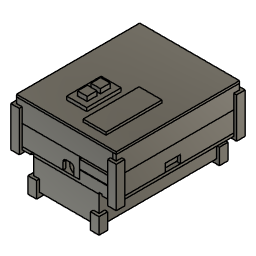
Thermocycler_build v6 (Autodesk Fusion 360 design; units mm, degrees)
Autodesk Fusion 360 part; units mm, degrees
(part 1 of 2)
sketch "Sketch1" plane through (0, 0, 0) normal (0, 0, 1) x (1, 0, 0)
  line L0 (0, 0) -> (114, 0)
  line L1 (114, 0) -> (114, 215)
  line L2 (114, 215) -> (0, 215)
  line L3 (0, 215) -> (0, 0)
  dimension "d1" = 114
  dimension "d2" = 215
  constraint horizontal L0
  constraint vertical L1
  constraint horizontal L2
  constraint vertical L3
  constraint coincident L0.start L3.end
  measures "d1" distance of L0.start L0.end
  measures "d2" distance of L0.start L2.end
extrude "Extrude1" add sketch "Sketch1" along normal blind 49 makes body 1
sketch "Sketch2" plane through (0, 0, 0) normal (0, 0, 1) x (1, 0, 0)
  line L0 (0, 0) -> (50, 0)
  line L1 (50, 0) -> (50, 138)
  line L2 (50, 138) -> (0, 138)
  line L3 (0, 138) -> (0, 0)
  dimension "d5" = 50
  dimension "d6" = 138
  constraint horizontal L0
  constraint vertical L1
  constraint horizontal L2
  constraint vertical L3
  constraint coincident L0.start L3.end
  measures "d5" distance of L0.start L0.end
  measures "d6" distance of L0.start L2.end
extrude "Extrude2" add sketch "Sketch2" along normal blind 21 separate body makes body 2
copy_body "Body->Comp1" bodies 1 removing the originals makes body 3 in component "Alimentatore"
copy_body "Body->Comp2" bodies 2 removing the originals makes body 4 in component "Relays"
sketch "Sketch3" plane through (0, 0, 0) normal (0, 0, 1) x (1, 0, 0)
  line L0 (0, 0) -> (26, 0)
  line L1 (26, 0) -> (26, 50)
  line L2 (26, 50) -> (0, 50)
  line L3 (0, 50) -> (0, 0)
  dimension "d9" = 26
  dimension "d10" = 50
  constraint horizontal L0
  constraint vertical L1
  constraint horizontal L2
  constraint vertical L3
  constraint coincident L0.start L3.end
  measures "d9" distance of L0.start L0.end
  measures "d10" distance of L0.start L2.end
extrude "Extrude3" add sketch "Sketch3" along normal blind 15 separate body makes body 5
copy_body "Body->Comp3" bodies 5 removing the originals makes body 6 in component "Buck_conv"
sketch "Sketch4" plane through (0, 0, 0) normal (0, 0, 1) x (1, 0, 0)
  line L0 (0, 0) -> (82, 0)
  line L1 (82, 0) -> (82, 54)
  line L2 (82, 54) -> (0, 54)
  line L3 (0, 54) -> (0, 0)
  dimension "d13" = 82
  dimension "d14" = 54
  constraint horizontal L0
  constraint vertical L1
  constraint horizontal L2
  constraint vertical L3
  constraint coincident L0.start L3.end
  measures "d13" distance of L0.start L0.end
  measures "d14" distance of L0.start L2.end
extrude "Extrude4" add sketch "Sketch4" along normal blind 10 separate body makes body 7
copy_body "Body->Comp4" bodies 7 removing the originals makes body 8 in component "Breadbord"
sketch "Sketch5" plane through (0, 0, 0) normal (0, 0, 1) x (1, 0, 0)
  line L0 (0, 0) -> (58, 0)
  line L1 (58, 0) -> (58, 82)
  line L2 (58, 82) -> (0, 82)
  line L3 (0, 82) -> (0, 0)
  dimension "d17" = 58
  dimension "d18" = 82
  constraint horizontal L0
  constraint vertical L1
  constraint horizontal L2
  constraint vertical L3
  constraint coincident L0.start L3.end
  measures "d17" distance of L0.start L0.end
  measures "d18" distance of L0.start L2.end
extrude "Extrude5" add sketch "Sketch5" along normal blind 15 separate body makes body 9
copy_body "Body->Comp5" bodies 9 removing the originals makes body 10 in component "Arduino"
sketch "Sketch6" plane through (0, 0, 0) normal (0, 0, 1) x (1, 0, 0)
  line L0 (0, 0) -> (18, 0)
  line L1 (18, 0) -> (18, 35)
  line L2 (18, 35) -> (0, 35)
  line L3 (0, 35) -> (0, 0)
  dimension "d21" = 18
  dimension "d22" = 35
  constraint horizontal L0
  constraint vertical L1
  constraint horizontal L2
  constraint vertical L3
  constraint coincident L0.start L3.end
  measures "d21" distance of L0.start L0.end
  measures "d22" distance of L0.start L2.end
extrude "Extrude6" add sketch "Sketch6" along normal blind 15 separate body makes body 11
copy_body "Body->Comp6" bodies 11 removing the originals makes body 12 in component "Mosfet"
sketch "Sketch7" plane through (0, 0, 0) normal (0, 0, 1) x (1, 0, 0)
  line L0 (0, 0) -> (40, 0)
  line L1 (40, 0) -> (40, 73)
  line L2 (40, 73) -> (0, 73)
  line L3 (0, 73) -> (0, 0)
  dimension "d25" = 40
  dimension "d26" = 73
  constraint horizontal L0
  constraint vertical L1
  constraint horizontal L2
  constraint vertical L3
  constraint coincident L0.start L3.end
  measures "d25" distance of L0.start L0.end
  measures "d26" distance of L0.start L2.end
extrude "Extrude7" add sketch "Sketch7" along normal blind 24 separate body makes body 13
copy_body "Body->Comp7" bodies 13 removing the originals makes body 14 in component "Big_relay"
copy_body "CopyPasteBodies1" bodies 12 makes body 15 in component "Mosfet"
move_body "Move1" bodies 15 to x (1, 0, 0) y (0, 1, 0) z (0, 0, 1) at (-20, 20, 0) in component "Mosfet"
move_body "Move2" bodies 12 to x (1, 0, 0) y (0, 1, 0) z (0, 0, 1) at (4, 0, 0) in component "Mosfet"
copy_body "CopyPasteBodies2" bodies 12 makes body 16 in component "Mosfet"
move_body "Move3" bodies 16 to x (1, 0, 0) y (0, 1, 0) z (0, 0, 1) at (0, 60, 0) in component "Mosfet"
sketch "Sketch8" plane through (0, 0, 49) normal (0, 0, 1) x (-1, 0, 0)
  line L0 (0, -215) -> (0, 0)
  line L1 (0, 0) -> (-114, 0)
  line L2 (-114, 0) -> (-114, -215)
  line L3 (-114, -215) -> (0, -215)
  line L4 (-144, 30) -> (-144, -245)
  line L5 (-144, -245) -> (30, -245)
  line L6 (30, -245) -> (30, 30)
  line L7 (30, 30) -> (-144, 30)
  line L8 (0, -215) -> (30, -215)
  line L9 (-114, -215) -> (-144, -215)
  line L10 (-114, 0) -> (-144, 0)
  line L11 (0, 0) -> (30, 0)
  line L12 (20, -203) -> (-30, -203)
  line L13 (-30, -203) -> (-30, -65)
  line L14 (-30, -65) -> (20, -65)
  line L15 (20, -65) -> (20, -203)
  line L16 (21.5, -51.5) -> (-51.5, -51.5)
  line L17 (-51.5, -51.5) -> (-51.5, -11.5)
  line L18 (-51.5, -11.5) -> (21.5, -11.5)
  line L19 (21.5, -11.5) -> (21.5, -51.5)
  line L20 (-36, -150) -> (-54, -150)
  line L21 (-54, -150) -> (-54, -115)
  line L22 (-54, -115) -> (-36, -115)
  line L23 (-36, -115) -> (-36, -150)
  line L24 (-60, -190) -> (-78, -190)
  line L25 (-78, -190) -> (-78, -155)
  line L26 (-78, -155) -> (-60, -155)
  line L27 (-60, -155) -> (-60, -190)
  line L28 (-36, -210) -> (-54, -210)
  line L29 (-54, -210) -> (-54, -175)
  line L30 (-54, -175) -> (-36, -175)
  line L31 (-36, -175) -> (-36, -210)
  line L32 (-88, -203) -> (-138, -203)
  line L33 (-138, -203) -> (-138, -177)
  line L34 (-138, -177) -> (-88, -177)
  line L35 (-88, -177) -> (-88, -203)
  line L36 (-84, -173) -> (-138, -173)
  line L37 (-138, -173) -> (-138, -91)
  line L38 (-138, -91) -> (-84, -91)
  line L39 (-84, -91) -> (-84, -173)
  line L40 (-80, -82) -> (-138, -82)
  line L41 (-138, -82) -> (-138, 0)
  line L42 (-138, 0) -> (-80, 0)
  line L43 (-80, 0) -> (-80, -82)
  line L44 (0, -215) -> (-114, -215)
  line L45 (-114, -215) -> (-114, 0)
  line L46 (-114, 0) -> (0, 0)
  line L47 (0, 0) -> (0, -215)
  line L48 (-114, 0) -> (-77, 0) construction
  line L49 (-77, 0) -> (-77, -44) construction
  line L50 (-77, -44) -> (-114, -44) construction
  line L51 (-114, -44) -> (-114, 0) construction
  circle A0 centre (-77, -44) radius 32.5
  line L52 (-80, 0) -> (-138, 0)
  line L53 (-138, 0) -> (-138, -9)
  line L54 (-138, -9) -> (-80, -9)
  line L55 (-80, -9) -> (-80, 0)
  line L56 (-138, -82) -> (-118, -82)
  line L57 (-118, -82) -> (-118, -72)
  line L58 (-118, -72) -> (-138, -72)
  line L59 (-138, -72) -> (-138, -82)
  dimension "d29" = 30
  dimension "d30" = 37
  dimension "d31" = 44
  dimension "d32" = 65
  dimension "d33" = 58
  dimension "d34" = 9
  dimension "d35" = 20
  dimension "d36" = 10
  constraint coincident L0.start L3.end
  constraint coincident L6 L8.end
  constraint perpendicular L6 L8
  constraint coincident L2.end L3.start
  constraint coincident L4 L9.end
  constraint perpendicular L4 L9
  constraint coincident L1.end L2.start
  constraint coincident L4 L10.end
  constraint perpendicular L4 L10
  constraint coincident L0.end L1.start
  constraint coincident L6 L11.end
  constraint perpendicular L6 L11
  constraint horizontal L12
  constraint vertical L13
  constraint horizontal L14
  constraint vertical L15
  constraint horizontal L16
  constraint vertical L17
  constraint horizontal L18
  constraint vertical L19
  constraint horizontal L20
  constraint vertical L21
  constraint horizontal L22
  constraint vertical L23
  constraint horizontal L24
  constraint vertical L25
  constraint horizontal L26
  constraint vertical L27
  constraint horizontal L28
  constraint vertical L29
  constraint horizontal L30
  constraint vertical L31
  constraint horizontal L32
  constraint vertical L33
  constraint horizontal L34
  constraint vertical L35
  constraint horizontal L36
  constraint vertical L37
  constraint horizontal L38
  constraint vertical L39
  constraint horizontal L40
  constraint vertical L41
  constraint horizontal L42
  constraint vertical L43
  constraint horizontal L44
  constraint vertical L45
  constraint horizontal L46
  constraint vertical L47
  constraint horizontal L48
  constraint vertical L49
  constraint horizontal L50
  constraint vertical L51
  constraint coincident L49.end L50.start
  constraint horizontal L52
  constraint vertical L53
  constraint horizontal L54
  constraint vertical L55
  constraint horizontal L56
  constraint vertical L57
  constraint horizontal L58
  constraint vertical L59
  measures "d30" distance of L1.end L48.end
  measures "d31" distance of L1.end L50.end
  measures "d32" diameter of A0
  measures "d33" distance of L42.end L41.end
  measures "d34" distance of L42.end L54.end
  measures "d35" distance of L40.end L56.end
  measures "d36" distance of L40.end L58.end
extrude "Extrude1'" add sketch "Sketch8" along normal blind 5 separate body contours L0 L2 L3 L12 L13 L14 L16 L32 L34 L35 L36 L38 L39 L40 L43 L44 L45 L47 A0 | L0 L6 L8 L11 L12 L14 L15 L16 L18 L19 L47 | L0 L12 L13 L14 L47 | L0 L12 L14 L15 L47 | L2 L4 L9 L10 L32 L33 L34 L36 L37 L38 L40 L41 L45 L53 L56 L59 | L2 L32 L33 L34 L45 | L2 L32 L34 L35 L45 | L0 L16 L17 L18 L47 A0 | L0 L16 L18 L19 L47 | L0 L1 L17 L18 L43 L46 L47 A0 L55 | L2 L36 L37 L38 L45 | L2 L36 L38 L39 L45 | L2 L10 L41 L42 L45 L52 L53 L54 | L1 L2 L42 L43 L45 L46 L52 L54 L55 | L2 L40 L43 L45 A0 L54 | L2 L40 L41 L45 L54 L57 L58 | L40 L41 L56 L57 L58 L59 | L20 L21 L22 L23 | L24 L25 L26 L27 | L28 L29 L30 L31 makes body 17 in component "Alimentatore"
copy_body "CutPasteBodies1" bodies 17 removing the originals makes body 18
extrude "Extrude8" add sketch "Sketch8" along normal blind 20 contours L2 L10 L41 L42 L45 L52 L53 L54 | L1 L2 L42 L43 L45 L46 L52 L54 L55 | L40 L41 L56 L57 L58 L59 bodies 18
fillet "Fillet1" radius 10 1 edges at (107.3006, 32.2475, 54) on bodies 18
sketch "Sketch9" plane through (0, 0, 54) normal (0, 0, 1) x (-1, 0, 0)
  arc A0 (-98.6603, -9) -> (-80, -2.9492) centre (-77, -44) ccw
  line L0 (-98.6603, -9) -> (-138, -9)
  line L1 (-138, -9) -> (-138, 0)
  line L2 (-138, 0) -> (-144, 0)
  line L3 (-144, 0) -> (-144, -215)
  line L4 (-144, -215) -> (30, -215)
  line L5 (30, -215) -> (30, 0)
  line L6 (30, 0) -> (-80, 0)
  line L7 (-80, 0) -> (-80, -2.9492)
  line L8 (-138, -72) -> (-118, -72)
  line L9 (-118, -72) -> (-118, -82)
  line L10 (-118, -82) -> (-138, -82)
  line L11 (-138, -82) -> (-138, -72)
  line L12 (-144, -215) -> (-114, -215) construction
  line L13 (30, -215) -> (0, -215) construction
  line L14 (-114, -215) -> (0, -215) construction
  line L15 (0, -215) -> (0, -195)
  line L16 (0, -195) -> (-114, -195)
  line L17 (-114, -195) -> (-114, -215)
  line L18 (-57, -195) -> (-57, -185) construction
  line L19 (-57, -185) -> (-47, -185) construction
  line L20 (-47, -185) -> (-22, -185) construction
  line L21 (-22, -185) -> (-47, -185)
  line L22 (-47, -185) -> (-47, -153)
  line L23 (-47, -153) -> (-22, -153)
  line L24 (-22, -153) -> (-22, -185)
  line L25 (-57, -185) -> (-82, -185)
  line L26 (-82, -185) -> (-82, -153)
  line L27 (-82, -153) -> (-57, -153)
  line L28 (-57, -153) -> (-57, -185)
  dimension "d43" = 30
  dimension "d44" = 30
  dimension "d45" = 20
  dimension "d46" = 10
  dimension "d47" = 10
  dimension "d48" = 25
  dimension "d49" = 25
  dimension "d50" = 32
  dimension "d51" = 25
  dimension "d52" = 32
  constraint coincident L3.end L4.start
  constraint perpendicular L3 L12
  constraint coincident L4.end L5.start
  constraint perpendicular L5 L13
  constraint horizontal L14
  constraint vertical L15
  constraint horizontal L16
  constraint vertical L17
  constraint midpoint L16 L18.start
  constraint perpendicular L16 L18
  constraint perpendicular L18 L19
  constraint parallel L19 L20
  constraint horizontal L21
  constraint vertical L22
  constraint horizontal L23
  constraint vertical L24
  constraint coincident L13.end L15
  constraint horizontal L25
  constraint vertical L26
  constraint horizontal L27
  constraint vertical L28
  measures "d43" distance of L3.end L12.end
  measures "d44" distance of L4.end L13.end
  measures "d45" distance of L12.end L16.end
  measures "d46" distance of L18.start L18.end
  measures "d47" distance of L18.end L19.end
  measures "d48" distance of L19.end L20.end
  measures "d49" distance of L20.end L19.end
  measures "d50" distance of L20.end L23.end
  measures "d51" distance of L18.end L25.end
  measures "d52" distance of L18.end L27.end
extrude "Extrude9" cut sketch "Sketch9" against normal blind 30 contours L4 L15 L16 L17 | L21 L22 L23 L24 | L25 L26 L27 L28 bodies 18
move_body "Move4" bodies 15 to x (1, 0, 0) y (0, 1, 0) z (0, 0, 1) at (0, 20, 0) in component "Mosfet"
move_body "Move5" bodies 12 to x (1, 0, 0) y (0, 1, 0) z (0, 0, 1) at (0, 35, 0) in component "Mosfet"
move_body "Move6" bodies 16 to x (1, 0, 0) y (0, 1, 0) z (0, 0, 1) at (0, 15, 0) in component "Mosfet"
move_body "Move7" bodies 15 to x (1, 0, 0) y (0, 1, 0) z (0, 0, 1) at (0, -10, 0) in component "Mosfet"
sketch "Sketch10" plane through (0, 0, 54) normal (0, 0, 1) x (-1, 0, 0)
  line L0 (0, -195) -> (0, -215)
  line L1 (0, -215) -> (30, -215)
  line L2 (30, -215) -> (30, 0)
  line L3 (30, 0) -> (-80, 0)
  line L4 (-80, 0) -> (-80, -2.9492)
  arc A0 (-98.6603, -9) -> (-80, -2.9492) centre (-77, -44) ccw
  line L5 (-98.6603, -9) -> (-138, -9)
  line L6 (-138, -9) -> (-138, 0)
  line L7 (-138, 0) -> (-144, 0)
  line L8 (-144, 0) -> (-144, -215)
  line L9 (-144, -215) -> (-114, -215)
  line L10 (-114, -215) -> (-114, -195)
  line L11 (-114, -195) -> (0, -195)
  line L12 (-82, -185) -> (-82, -153)
  line L13 (-82, -153) -> (-57, -153)
  line L14 (-57, -153) -> (-57, -185)
  line L15 (-57, -185) -> (-82, -185)
  line L16 (-47, -185) -> (-47, -153)
  line L17 (-47, -153) -> (-22, -153)
  line L18 (-22, -153) -> (-22, -185)
  line L19 (-22, -185) -> (-47, -185)
  line L20 (-138, -72) -> (-118, -72)
  line L21 (-118, -72) -> (-118, -82)
  line L22 (-118, -82) -> (-138, -82)
  line L23 (-138, -82) -> (-138, -72)
  line L24 (0, -210) -> (25, -210)
  line L25 (25, -210) -> (25, -5)
  line L26 (25, -5) -> (-80, -5)
  line L27 (-138, -5) -> (-139, -5)
  line L28 (-139, -5) -> (-139, -210)
  line L29 (-139, -210) -> (-114, -210)
  line L30 (-138, -5) -> (-138, 0)
  line L31 (-114, -210) -> (-114, -215)
  line L32 (-114, -210) -> (0, -210)
  line L33 (-114, -215) -> (0, -215)
  line L34 (-80, -5) -> (-80, 0)
  dimension "d55" = -5
  dimension "d56" = -5
  constraint coincident L6.end L7.start
  constraint perpendicular L7 L30
  constraint coincident L9.end L10.start
  constraint perpendicular L9 L31
  constraint perpendicular L0 L32
  constraint coincident L0.end L1.start
  constraint coincident L3.end L4.start
  constraint perpendicular L3 L34
extrude "Extrude10" add sketch "Sketch10" along normal blind 35 separate body contours L0 L1 L2 L3 L4 A0 L24 L25 L26 L34 | L0 L10 L31 L32 L33 | L6 L7 L8 L9 L10 L27 L28 L29 L30 L31 | A0 L26 L34 makes body 19
extrude "Extrude11" add 1 faces at (37.9469, 1.6667, 89) along direction (0, 0, 1) blind 40 separate body on bodies 19 makes body 20
extrude "Extrude12" add 2 faces at (80, 0.9831, 102.3333) (80, 4.3164, 102.3333) along direction (1, 0, 0) blind 60 on bodies 20 bodies 20
sketch "Sketch11" plane through (0, 0, 0) normal (0, 0, 1) x (1, 0, 0)
  line L0 (0, 0) -> (100, 0)
  line L1 (100, 0) -> (100, 60)
  line L2 (100, 60) -> (0, 60)
  line L3 (0, 60) -> (0, 0)
  line L4 (98.75, 10.1) -> (1.25, 10.1)
  line L5 (1.25, 10.1) -> (1.25, 49.9)
  line L6 (1.25, 49.9) -> (98.75, 49.9)
  line L7 (98.75, 49.9) -> (98.75, 10.1)
  line L8 (98.75, 10.1) -> (1.25, 49.9) construction
  line L9 (1.25, 10.1) -> (98.75, 49.9) construction
  point P0 (50, 30)
  dimension "d63" = 100
  dimension "d64" = 60
  dimension "d65" = 39.8
  dimension "d66" = 97.5
  dimension "d67" = 50
  dimension "d68" = 30
  constraint horizontal L0
  constraint vertical L1
  constraint horizontal L2
  constraint vertical L3
  constraint coincident L0.start L3.end
  constraint horizontal L4
  constraint perpendicular L4 L5
  constraint parallel L4 L6
  constraint parallel L5 L7
  constraint coincident L8 P0
  constraint coincident L9 P0
  measures "d63" distance of L0.start L0.end
  measures "d64" distance of L0.start L2.end
  measures "d65" distance of L4.end L5.end
  measures "d66" distance of L5.end L6.end
  measures "d67" distance of L1 P0
  measures "d68" distance of L2 P0
extrude "Extrude13" add sketch "Sketch11" along normal blind 2 separate body makes body 21
extrude "Extrude14" add sketch "Sketch11" along normal blind 10.5 contours L4 L5 L6 L7 bodies 21
move_body "Move1'" bodies 21 to x (0, -1, 0) y (1, 0, 0) z (0, 0, 1) at (-20, 110, 127)
sketch "Sketch12" plane through (0, 0, 129) normal (0, 0, 1) x (-1, 0, 0)
  line L0 (-138, -5) -> (25, -5)
  line L1 (25, -5) -> (25, -210)
  line L2 (25, -210) -> (-139, -210)
  line L3 (-139, -210) -> (-139, -5)
  line L4 (-139, -5) -> (-138, -5)
  line L5 (30, 0) -> (-138, 0)
  line L6 (-138, 0) -> (-144, 0)
  line L7 (-144, 0) -> (-144, -215)
  line L8 (-144, -215) -> (30, -215)
  line L9 (30, -215) -> (30, 0)
  line L10 (-144, 0) -> (30, 0)
  line L11 (30, 0) -> (30, -215)
  line L12 (30, -215) -> (-144, -215)
  line L13 (-144, -215) -> (-144, 0)
  line L14 (-119.9, -15) -> (-59.9, -15) construction
  line L15 (-59.9, -15) -> (-59.9, -115) construction
  line L16 (-59.9, -115) -> (-119.9, -115) construction
  line L17 (-119.9, -115) -> (-119.9, -15) construction
  line L18 (-119.9, -65) -> (-59.9, -65) construction
  line L19 (-89.9, -15) -> (-89.9, -115) construction
  line L20 (-69.9, -113.75) -> (-109.9, -113.75)
  line L21 (-109.9, -113.75) -> (-109.9, -16.25)
  line L22 (-109.9, -16.25) -> (-69.9, -16.25)
  line L23 (-69.9, -16.25) -> (-69.9, -113.75)
  line L24 (-69.9, -113.75) -> (-109.9, -16.25) construction
  line L25 (-109.9, -113.75) -> (-69.9, -16.25) construction
  point P0 (-89.9, -65)
  dimension "d73" = 40
  dimension "d74" = 97.5
  constraint horizontal L10
  constraint vertical L11
  constraint horizontal L12
  constraint vertical L13
  constraint coincident L8.end L9.start
  constraint coincident L6.end L7.start
  constraint horizontal L14
  constraint vertical L15
  constraint horizontal L16
  constraint vertical L17
  constraint midpoint L17 L18.start
  constraint midpoint L15 L18.end
  constraint midpoint L14 L19.start
  constraint midpoint L16 L19.end
  constraint horizontal L20
  constraint perpendicular L20 L21
  constraint parallel L20 L22
  constraint parallel L21 L23
  constraint coincident L24 P0
  constraint coincident L25 P0
  constraint midpoint L18 P0
  measures "d73" distance of L21.end L22.end
  measures "d74" distance of L20.end L21.end
extrude "Extrude15" add sketch "Sketch12" along normal blind 5 separate body contours L0 L1 L2 L3 L4 | L5 L6 L7 L8 L9 L10 L11 L12 L13 makes body 22
sketch "Sketch13" plane through (0, 0, 49) normal (0, 0, -1) x (1, 0, 0)
  circle A0 centre (77, -44) radius 32.5
  line L0 (0, -215) -> (0, -195)
  line L1 (0, -195) -> (114, -195)
  line L2 (114, -195) -> (114, -215)
  line L3 (114, -215) -> (144, -215)
  line L4 (144, -215) -> (144, 0)
  line L5 (144, 0) -> (-30, 0)
  line L6 (-30, 0) -> (-30, -215)
  line L7 (-30, -215) -> (0, -215)
  line L8 (47, -153) -> (47, -185)
  line L9 (47, -185) -> (22, -185)
  line L10 (22, -185) -> (22, -153)
  line L11 (22, -153) -> (47, -153)
  line L12 (82, -153) -> (82, -185)
  line L13 (82, -185) -> (57, -185)
  line L14 (57, -185) -> (57, -153)
  line L15 (57, -153) -> (82, -153)
  line L16 (0, 0) -> (-5, 0)
  line L17 (-5, 0) -> (-5, -215)
  line L18 (-5, -215) -> (0, -215)
  line L19 (0, -215) -> (0, 0)
  line L20 (114, 0) -> (119, 0)
  line L21 (119, 0) -> (119, -215)
  line L22 (119, -215) -> (114, -215)
  line L23 (114, -215) -> (114, 0)
  dimension "d77" = 5
  constraint horizontal L16
  constraint vertical L17
  constraint horizontal L18
  constraint vertical L19
  constraint coincident L7 L17.end
  constraint coincident L16.start L19.end
  constraint horizontal L20
  constraint vertical L21
  constraint horizontal L22
  constraint vertical L23
  constraint coincident L3 L21.end
  constraint coincident L5 L20.start
  measures "d77" distance of L20.start L20.end
extrude "Extrude16" cut sketch "Sketch13" against normal blind 2.5 contours L0 L5 L7 L16 L17 L18 L19 | L2 L3 L5 L20 L21 L22 L23 bodies 18
sketch "Sketch14" plane through (0, 0, 0) normal (0, -1, 0) x (1, 0, 0)
  line L0 (-30, 54) -> (80, 54)
  line L1 (80, 54) -> (80, 89)
  line L2 (80, 89) -> (-30, 89)
  line L3 (-30, 89) -> (-30, 54)
  line L4 (70, 54) -> (51, 54)
  line L5 (51, 54) -> (51, 66.5)
  line L6 (56.5, 72) -> (64.5, 72)
  line L7 (70, 66.5) -> (70, 54)
  arc A0 (56.5, 72) -> (51, 66.5) centre (56.5, 66.5) ccw
  arc A1 (70, 66.5) -> (64.5, 72) centre (64.5, 66.5) ccw
  point P0 (70, 72)
  dimension "d80" = 19
  dimension "d81" = 18
  dimension "d82" = 5.5
  constraint horizontal L4
  constraint vertical L5
  constraint horizontal L6
  constraint vertical L7
  constraint coincident L0 L4.start
  constraint tangent L5 A0
  constraint tangent L6 A0
  constraint coincident P0 L6
  constraint coincident P0 L7
  constraint tangent L6 A1
  constraint tangent L7 A1
  constraint equal A0 A1
  measures "d80" distance of L4.start L4.end
  measures "d81" distance of L4.start P0
  measures "d82" radius of A0
extrude "Extrude17" cut sketch "Sketch14" against normal blind 10 contours L0 L4 L5 L6 L7 A0 A1 bodies 19
sketch "Sketch15" plane through (144, 0, 0) normal (1, 0, 0) x (0, 1, 0)
  line L0 (0, 54) -> (215, 54)
  line L1 (215, 54) -> (215, 89)
  line L2 (215, 89) -> (0, 89)
  line L3 (0, 89) -> (0, 54)
  line L4 (0, 89) -> (82, 89)
  line L5 (82, 89) -> (82, 89)
  line L6 (82, 89) -> (0, 89)
  line L7 (0, 89) -> (0, 89)
  line L8 (82, 89) -> (85.5, 89) construction
  line L9 (85.5, 89) -> (85.5, 54) construction
  line L10 (85.5, 54) -> (112, 54)
  line L11 (112, 54) -> (112, 68)
  line L12 (112, 68) -> (85.5, 68)
  line L13 (85.5, 68) -> (85.5, 54)
  dimension "d85" = 3.5
  dimension "d86" = 26.5
  dimension "d87" = 14
  constraint horizontal L4
  constraint horizontal L6
  constraint coincident L2 L4.end
  constraint coincident L2.end L3.start
  constraint parallel L2 L8
  constraint coincident L0 L9.end
  constraint perpendicular L0 L9
  constraint horizontal L10
  constraint vertical L11
  constraint horizontal L12
  constraint vertical L13
  measures "d85" distance of L4.end L8.end
  measures "d86" distance of L9.end L10.end
  measures "d87" distance of L9.end L12.end
extrude "Extrude18" cut sketch "Sketch15" against normal blind 5 contours L0 L10 L11 L12 L13 bodies 19
sketch "Sketch16" plane through (0, 215, 0) normal (0, 1, 0) x (-1, 0, 0)
  line L0 (-144, 54) -> (30, 54)
  line L1 (30, 54) -> (30, 89)
  line L2 (30, 89) -> (-144, 89)
  line L3 (-144, 89) -> (-144, 54)
  circle A0 centre (-119.9965, 81.996) radius 2.5
  circle A1 centre (-105, 65) radius 2.5
  line L4 (-103.1254, 66.6541) -> (-118.1219, 83.6501)
  line L5 (-121.8711, 80.342) -> (-106.8746, 63.3459)
  circle A2 centre (-104.2822, 81.996) radius 2.5
  circle A3 centre (-89.2857, 65) radius 2.5
  line L6 (-106.1568, 80.342) -> (-91.1603, 63.3459)
  line L7 (-87.4111, 66.6541) -> (-102.4076, 83.6501)
  circle A4 centre (-88.5679, 81.996) radius 2.5
  circle A5 centre (-73.5714, 65) radius 2.5
  line L8 (-90.4425, 80.342) -> (-75.446, 63.3459)
  line L9 (-71.6968, 66.6541) -> (-86.6933, 83.6501)
  circle A6 centre (-72.8536, 81.996) radius 2.5
  circle A7 centre (-57.8571, 65) radius 2.5
  line L10 (-74.7282, 80.342) -> (-59.7317, 63.3459)
  line L11 (-55.9825, 66.6541) -> (-70.979, 83.6501)
  circle A8 centre (-57.1393, 81.996) radius 2.5
  circle A9 centre (-42.1429, 65) radius 2.5
  line L12 (-59.0139, 80.342) -> (-44.0175, 63.3459)
  line L13 (-40.2683, 66.6541) -> (-55.2647, 83.6501)
  circle A10 centre (-41.425, 81.996) radius 2.5
  circle A11 centre (-26.4286, 65) radius 2.5
  line L14 (-43.2996, 80.342) -> (-28.3032, 63.3459)
  line L15 (-24.554, 66.6541) -> (-39.5505, 83.6501)
  circle A12 centre (-25.7108, 81.996) radius 2.5
  circle A13 centre (-10.7143, 65) radius 2.5
  line L16 (-27.5854, 80.342) -> (-12.5889, 63.3459)
  line L17 (-8.8397, 66.6541) -> (-23.8362, 83.6501)
  circle A14 centre (-9.9965, 81.996) radius 2.5
  circle A15 centre (5, 65) radius 2.5
  line L18 (-11.8711, 80.342) -> (3.1254, 63.3459)
  line L19 (6.8746, 66.6541) -> (-8.1219, 83.6501)
  dimension "d90" = 5
  dimension "d91" = 5
  dimension "d94" = 110
  dimension "d95" = 0
  constraint coincident A1 L4.start
  constraint coincident A0 L4.end
  constraint tangent A0 L4
  constraint coincident A0 L5.start
  constraint coincident A1 L5.end
  constraint tangent A1 L5
  constraint tangent A1 L4
  constraint tangent A0 L5
  measures "d90" diameter of A0
  measures "d91" diameter of A1
extrude "Extrude19" cut sketch "Sketch16" against normal blind 5 contours A0 | A0 A1 L4 L5 | A1 | A2 | A2 A3 L6 L7 | A3 | A4 | A4 A5 L8 L9 | A5 | A6 | A6 A7 L10 L11 | A7 | A8 | A8 A9 L12 L13 | A9 | A10 | A10 A11 L14 L15 | A11 | A12 | A12 A13 L16 L17 | A13 | A14 | A14 A15 L18 L19 | A15 bodies 19
move_face "OffsetFaces1" offset -5 1 faces at (-28.3333, 73.3333, 129) on bodies 20
sketch "Sketch17" plane through (0, 0, 124) normal (0, 0, 1) x (-1, 0, 0)
  line L0 (-138, -5) -> (25, -5)
  line L1 (25, -5) -> (25, -210)
  line L2 (25, -210) -> (-139, -210)
  line L3 (-139, -210) -> (-139, -5)
  line L4 (-139, -5) -> (-138, -5)
  line L5 (30, 0) -> (-138, 0)
  line L6 (-138, 0) -> (-144, 0)
  line L7 (-144, 0) -> (-144, -215)
  line L8 (-144, -215) -> (30, -215)
  line L9 (30, -215) -> (30, 0)
  line L10 (25, -210) -> (10, -210)
  line L11 (10, -210) -> (10, -195)
  line L12 (10, -195) -> (25, -195)
  line L13 (25, -195) -> (25, -210)
  line L14 (-124, -195) -> (-139, -195)
  line L15 (-139, -195) -> (-139, -210)
  line L16 (-139, -210) -> (-124, -210)
  line L17 (-124, -210) -> (-124, -195)
  line L18 (25, -5) -> (10, -5)
  line L19 (10, -5) -> (10, -20)
  line L20 (10, -20) -> (25, -20)
  line L21 (25, -20) -> (25, -5)
  line L22 (-139, -5) -> (-124, -5)
  line L23 (-124, -5) -> (-124, -20)
  line L24 (-124, -20) -> (-139, -20)
  line L25 (-139, -20) -> (-139, -5)
  line L26 (10, -100) -> (40, -100)
  line L27 (40, -100) -> (40, -115)
  line L28 (40, -115) -> (10, -115)
  line L29 (10, -115) -> (10, -100)
  line L30 (10, -100) -> (40, -115) construction
  line L31 (40, -100) -> (10, -115) construction
  line L32 (-64.5, -195) -> (-49.5, -195)
  line L33 (-49.5, -195) -> (-49.5, -225)
  line L34 (-49.5, -225) -> (-64.5, -225)
  line L35 (-64.5, -225) -> (-64.5, -195)
  line L36 (-64.5, -195) -> (-49.5, -225) construction
  line L37 (-49.5, -195) -> (-64.5, -225) construction
  line L38 (-154, -100) -> (-124, -100)
  line L39 (-124, -100) -> (-124, -115)
  line L40 (-124, -115) -> (-154, -115)
  line L41 (-154, -115) -> (-154, -100)
  line L42 (-154, -100) -> (-124, -115) construction
  line L43 (-124, -100) -> (-154, -115) construction
  line L44 (-64, 10) -> (-49, 10)
  line L45 (-49, 10) -> (-49, -20)
  line L46 (-49, -20) -> (-64, -20)
  line L47 (-64, -20) -> (-64, 10)
  line L48 (-64, 10) -> (-49, -20) construction
  line L49 (-49, 10) -> (-64, -20) construction
  line L50 (25, -20) -> (10, -20)
  line L51 (10, -20) -> (10, -40)
  line L52 (10, -40) -> (25, -40)
  line L53 (25, -40) -> (25, -20)
  line L54 (-124, -20) -> (-139, -20)
  line L55 (10, -5) -> (-10, -5)
  line L56 (-10, -5) -> (-10, -20)
  line L57 (-10, -20) -> (10, -20)
  line L58 (10, -20) -> (10, -5)
  line L59 (-139, -195) -> (-124, -195)
  line L60 (-124, -195) -> (-124, -175)
  line L61 (-124, -175) -> (-139, -175)
  line L62 (-139, -175) -> (-139, -195)
  line L63 (-124, -195) -> (-104, -195)
  line L64 (-104, -195) -> (-104, -210)
  line L65 (-104, -210) -> (-124, -210)
  line L66 (-124, -210) -> (-124, -195)
  line L67 (-44.5, -190) -> (-69.5, -190)
  line L68 (-69.5, -190) -> (-69.5, -210)
  line L69 (-69.5, -210) -> (-44.5, -210)
  line L70 (-44.5, -210) -> (-44.5, -190)
  line L71 (25, -195) -> (10, -195)
  line L72 (10, -195) -> (10, -175)
  line L73 (10, -175) -> (25, -175)
  line L74 (25, -175) -> (25, -195)
  line L75 (10, -195) -> (-10, -195)
  line L76 (-10, -195) -> (-10, -210)
  line L77 (-10, -210) -> (10, -210)
  line L78 (10, -210) -> (10, -195)
  line L79 (30, -215) -> (-144, 0) construction
  line L80 (5, -95) -> (25, -95)
  line L81 (25, -95) -> (25, -120)
  line L82 (25, -120) -> (5, -120)
  line L83 (5, -120) -> (5, -95)
  point P0 (25, -107.5)
  point P1 (-57, -210)
  point P2 (-139, -107.5)
  point P3 (-56.5, -5)
  dimension "d99" = 15
  dimension "d100" = 15
  dimension "d101" = 15
  dimension "d102" = 15
  dimension "d103" = 15
  dimension "d104" = 15
  dimension "d105" = 15
  dimension "d106" = 15
  dimension "d107" = 30
  dimension "d108" = 15
  dimension "d109" = 15
  dimension "d110" = 30
  dimension "d111" = 30
  dimension "d112" = 15
  dimension "d113" = 15
  dimension "d114" = 30
  dimension "d121" = 15
  dimension "d122" = 5
  dimension "d123" = 5
  dimension "d124" = 5
  dimension "d125" = 5
  constraint horizontal L10
  constraint vertical L11
  constraint horizontal L12
  constraint vertical L13
  constraint coincident L1.end L2.start
  constraint horizontal L14
  constraint vertical L15
  constraint horizontal L16
  constraint vertical L17
  constraint coincident L2.end L3.start
  constraint horizontal L18
  constraint vertical L19
  constraint horizontal L20
  constraint vertical L21
  constraint coincident L0.end L1.start
  constraint horizontal L22
  constraint vertical L23
  constraint horizontal L24
  constraint vertical L25
  constraint coincident L3.end L4.start
  constraint horizontal L26
  constraint perpendicular L26 L27
  constraint parallel L26 L28
  constraint parallel L27 L29
  constraint coincident L30 P0
  constraint coincident L31 P0
  constraint midpoint L1 P0
  constraint horizontal L32
  constraint perpendicular L32 L33
  constraint parallel L32 L34
  constraint parallel L33 L35
  constraint coincident L36 P1
  constraint coincident L37 P1
  constraint midpoint L2 P1
  constraint horizontal L38
  constraint perpendicular L38 L39
  constraint parallel L38 L40
  constraint parallel L39 L41
  constraint coincident L42 P2
  constraint coincident L43 P2
  constraint midpoint L3 P2
  constraint horizontal L44
  constraint perpendicular L44 L45
  constraint parallel L44 L46
  constraint parallel L45 L47
  constraint coincident L48 P3
  constraint coincident L49 P3
  constraint midpoint L0 P3
  constraint horizontal L50
  constraint vertical L51
  constraint horizontal L52
  constraint vertical L53
  constraint horizontal L54
  constraint horizontal L55
  constraint vertical L56
  constraint horizontal L57
  constraint vertical L58
  constraint horizontal L59
  constraint vertical L60
  constraint horizontal L61
  constraint vertical L62
  constraint horizontal L63
  constraint vertical L64
  constraint horizontal L65
  constraint vertical L66
  constraint coincident L2 L64.end
  constraint horizontal L67
  constraint vertical L68
  constraint horizontal L69
  constraint vertical L70
  constraint coincident L2 L68.end
  constraint horizontal L71
  constraint vertical L72
  constraint horizontal L73
  constraint vertical L74
  constraint horizontal L75
  constraint vertical L76
  constraint horizontal L77
  constraint vertical L78
  constraint coincident L2 L76.end
  constraint coincident L8.end L9.start
  constraint coincident L6.end L7.start
  constraint horizontal L80
  constraint vertical L81
  constraint horizontal L82
  constraint vertical L83
  constraint coincident L1 L81.end
  measures "d99" distance of L14.start L16.end
  measures "d100" distance of L14.start L14.end
  measures "d101" distance of L11.end L12.end
  measures "d102" distance of L3.end L22.end
  measures "d103" distance of L3.end L24.end
  measures "d104" distance of L10.end L11.end
  measures "d105" distance of L19.end L20.end
  measures "d106" distance of L18.end L19.end
  measures "d107" distance of L27.end L28.end
  measures "d108" distance of L26.end L27.end
  measures "d109" distance of L33.end L34.end
  measures "d110" distance of L32.end L33.end
  measures "d111" distance of L39.end L40.end
  measures "d112" distance of L38.end L39.end
  measures "d113" distance of L45.end L46.end
  measures "d114" distance of L44.end L45.end
  measures "d121" distance of L60 L62
  measures "d122" distance of L35 L68
  measures "d123" distance of L33 L70
  measures "d124" distance of L28 L82
  measures "d125" distance of L26 L80
extrude "Extrude20" add sketch "Sketch17" against normal blind 6 contours L0 L3 L4 L22 L23 L24 L25 L54 | L0 L45 L46 L47 | L3 L38 L39 L40 | L0 L1 L18 L19 L20 L21 L50 L58 | L2 L3 L14 L15 L16 L17 L59 L66 | L1 L26 L28 L29 L81 | L2 L32 L33 L35 L69 | L1 L2 L10 L11 L12 L13 L71 L78 bodies 20
sketch "Sketch18" plane through (0, 0, 134) normal (0, 0, 1) x (-1, 0, 0)
  line L0 (-109.9, -16.25) -> (-69.9, -16.25)
  line L1 (-69.9, -16.25) -> (-69.9, -113.75)
  line L2 (-69.9, -113.75) -> (-109.9, -113.75)
  line L3 (-109.9, -113.75) -> (-109.9, -16.25)
  line L4 (-144, -215) -> (30, -215)
  line L5 (30, -215) -> (30, 0)
  line L6 (30, 0) -> (-144, 0)
  line L7 (-144, 0) -> (-144, -215)
  line L8 (-69.9, -65) -> (30, -65) construction
  line L9 (-27.5, -40) -> (-52.5, -40)
  line L10 (-52.5, -40) -> (-52.5, -90)
  line L11 (-52.5, -90) -> (-27.5, -90)
  line L12 (-27.5, -90) -> (-27.5, -40)
  line L13 (-27.5, -40) -> (-52.5, -90) construction
  line L14 (-52.5, -40) -> (-27.5, -90) construction
  point P0 (-40, -65)
  dimension "d117" = 25
  dimension "d118" = 50
  constraint midpoint L1 L8.start
  constraint perpendicular L1 L8
  constraint horizontal L9
  constraint perpendicular L9 L10
  constraint parallel L9 L11
  constraint parallel L10 L12
  constraint coincident L13 P0
  constraint coincident L14 P0
  constraint coincident L8 P0
  measures "d117" distance of L10.end L11.end
  measures "d118" distance of L9.end L10.end
extrude "Extrude21" cut sketch "Sketch18" against normal blind 10 contours L9 L10 L11 L12 bodies 22
extrude "Extrude22" add sketch "Sketch17" along normal blind 10 contours L0 L19 L55 L56 L57 L58 | L3 L14 L59 L60 L61 L62 | L1 L20 L50 L51 L52 L53 | L1 L26 L28 L29 L80 L81 L82 L83 | L2 L17 L63 L64 L65 L66 | L2 L32 L33 L35 L67 L68 L69 L70 | L1 L12 L71 L72 L73 L74 | L2 L11 L75 L76 L77 L78 bodies 22
move_face "OffsetFaces2" offset -1 1 faces at (61.3, 181.25, 134) on bodies 22
sketch "Sketch1 (2)" plane through (0, 0, 0) normal (0, 0, 1) x (1, 0, 0) in component "Switch_holder"
  line L0 (0, 0) -> (-50, 0)
  line L1 (-50, 0) -> (-50, -25)
  line L2 (-50, -25) -> (0, -25)
  line L3 (0, -25) -> (0, 0)
  line L4 (0, -12.5) -> (-50, -12.5) construction
  line L5 (-22.15, -4) -> (-4.65, -4)
  line L6 (-4.65, -4) -> (-4.65, -21)
  line L7 (-4.65, -21) -> (-22.15, -21)
  line L8 (-22.15, -21) -> (-22.15, -4)
  line L9 (-22.15, -4) -> (-4.65, -21) construction
  line L10 (-4.65, -4) -> (-22.15, -21) construction
  line L11 (-25, -25) -> (-25, 0) construction
  line L12 (-45.35, -21) -> (-27.85, -21)
  line L13 (-45.35, -4) -> (-45.35, -21)
  line L14 (-27.85, -4) -> (-45.35, -4)
  line L15 (-27.85, -21) -> (-27.85, -4)
  line L16 (-22.15, -21) -> (-23, -21)
  line L17 (-23, -21) -> (-23, -4)
  line L18 (-23, -4) -> (-22.15, -4)
  line L19 (-22.15, -4) -> (-22.15, -21) construction
  line L20 (-27.85, -21) -> (-27, -21)
  line L21 (-27, -21) -> (-27, -4)
  line L22 (-27, -4) -> (-27.85, -4)
  line L23 (-27.85, -4) -> (-27.85, -21) construction
  line L24 (-50, 0) -> (-55, 0)
  line L25 (-55, 0) -> (-55, -25)
  line L26 (-55, -25) -> (-50, -25)
  line L27 (-50, -25) -> (-50, 0)
  line L28 (0, 0) -> (5, 0)
  line L29 (5, 0) -> (5, -25)
  line L30 (5, -25) -> (0, -25)
  line L31 (0, -25) -> (0, 0)
  point P0 (-13.4, -12.5)
  dimension "d129" = 50
  dimension "d130" = 25
  dimension "d131" = 17.5
  dimension "d132" = 17
  dimension "d133" = 5.7
  constraint horizontal L0
  constraint vertical L1
  constraint horizontal L2
  constraint vertical L3
  constraint coincident L0.start L3.end
  constraint midpoint L3 L4.start
  constraint midpoint L1 L4.end
  constraint horizontal L5
  constraint perpendicular L5 L6
  constraint parallel L5 L7
  constraint parallel L6 L8
  constraint coincident L9 P0
  constraint coincident L10 P0
  constraint coincident L4 P0
  constraint midpoint L2 L11.start
  constraint midpoint L0 L11.end
  constraint symmetric L5.start L11 L14.start
  constraint symmetric L5.end L11 L13.start
  constraint symmetric L6.end L11 L12.start
  constraint symmetric L7.end L11 L12.end
  constraint horizontal L16
  constraint vertical L17
  constraint horizontal L18
  constraint vertical L19
  constraint horizontal L20
  constraint vertical L21
  constraint horizontal L22
  constraint vertical L23
  constraint horizontal L24
  constraint vertical L25
  constraint horizontal L26
  constraint vertical L27
  constraint horizontal L28
  constraint vertical L29
  constraint horizontal L30
  constraint vertical L31
  measures "d129" distance of L1 L3
  measures "d130" distance of L0 L2
  measures "d131" distance of L6.end L7.end
  measures "d132" distance of L5.end L6.end
  measures "d133" distance of L8 L15
extrude "Extrude1''" add sketch "Sketch1 (2)" against normal blind 2 separate body contours L0 L1 L2 L3 L27 L31 | L5 L6 L7 L8 | L8 L16 L17 L18 | L12 L13 L14 L15 | L15 L20 L21 L22 makes body 23 in component "Switch_holder"
extrude "Extrude2'" add sketch "Sketch1 (2)" along normal blind 6.5 contours L0 L1 L2 L3 L27 L31 bodies 23 in component "Switch_holder"
sketch "Sketch2 (2)" plane through (0, 0, 6.5) normal (0, 0, 1) x (-1, 0, 0) in component "Switch_holder"
  line L0 (23, 21) -> (23, 4)
  line L1 (23, 4) -> (4.65, 4)
  line L2 (4.65, 4) -> (4.65, 21)
  line L3 (4.65, 21) -> (23, 21)
  line L4 (45.35, 4) -> (27, 4)
  line L5 (27, 4) -> (27, 21)
  line L6 (27, 21) -> (45.35, 21)
  line L7 (45.35, 21) -> (45.35, 4)
  line L8 (0, 25) -> (0, 0)
  line L9 (0, 0) -> (50, 0)
  line L10 (50, 0) -> (50, 25)
  line L11 (50, 25) -> (0, 25)
  line L12 (50, 0) -> (45.35, 0)
  line L13 (45.35, 0) -> (45.35, 25)
  line L14 (45.35, 25) -> (50, 25)
  line L15 (50, 25) -> (50, 0)
  line L16 (0, 0) -> (4.65, 0)
  line L17 (4.65, 0) -> (4.65, 25)
  line L18 (4.65, 25) -> (0, 25)
  line L19 (0, 25) -> (0, 0)
  constraint horizontal L12
  constraint vertical L13
  constraint horizontal L14
  constraint vertical L15
  constraint coincident L11 L13.end
  constraint coincident L9.end L10.start
  constraint horizontal L16
  constraint vertical L17
  constraint horizontal L18
  constraint vertical L19
  constraint coincident L11 L17.end
  constraint coincident L8.end L9.start
extrude "Extrude3'" add sketch "Sketch1 (2)" along normal blind 23 contours L3 L28 L29 L30 L31 | L1 L24 L25 L26 L27 bodies 23 in component "Switch_holder"
sketch "Sketch3 (2)" plane through (0, 0, 0) normal (1, 0, 0) x (0, 1, 0) in component "Switch_holder"
  line L0 (-25, 0) -> (-25, -2)
  line L1 (-25, -2) -> (0, -2)
  line L2 (0, -2) -> (0, 0)
  line L3 (-25, 0) -> (0, 0)
  line L4 (0, 0) -> (0, 18)
  line L5 (0, 18) -> (-25, 18)
  line L6 (-25, 18) -> (-25, 0)
  line L7 (0, 0) -> (-25, 0)
  constraint horizontal L3
  constraint vertical L4
  constraint horizontal L5
  constraint vertical L6
  constraint coincident L2 L4.end
  constraint coincident L0.start L3.start
sketch "Sketch4 (2)" plane through (0, 0, 6.5) normal (0, 0, 1) x (-1, 0, 0) in component "Switch_holder"
  line L0 (4.65, 21) -> (23, 21)
  line L1 (23, 21) -> (23, 4)
  line L2 (23, 4) -> (4.65, 4)
  line L3 (4.65, 4) -> (4.65, 21)
  line L4 (0, 0) -> (50, 0)
  line L5 (45.35, 4) -> (27, 4)
  line L6 (27, 4) -> (27, 21)
  line L7 (27, 21) -> (45.35, 21)
  line L8 (45.35, 21) -> (45.35, 4)
  line L9 (50, 25) -> (0, 25)
  line L10 (25, 0) -> (25, 25) construction
  line L11 (0, 25) -> (0, 0)
  line L12 (50, 0) -> (50, 25)
  constraint midpoint L4 L10.start
  constraint perpendicular L4 L10
extrude "Extrude4'" add sketch "Sketch1 (2)" against normal up to surface (2 mm away) contours L3 L28 L29 L30 L31 | L1 L24 L25 L26 L27 bodies 23 in component "Switch_holder"
sketch "Sketch5 (2)" plane through (0, 0, 6.5) normal (0, 0, 1) x (-1, 0, 0) in component "Switch_holder"
  line L0 (55, -5) -> (-5, -5)
  line L1 (-5, -5) -> (-5, 30)
  line L2 (-5, 30) -> (55, 30)
  line L3 (55, 30) -> (55, -5)
  line L4 (45.35, 4) -> (27.85, 4)
  line L5 (27.85, 4) -> (27.85, 21)
  line L6 (27.85, 21) -> (45.35, 21)
  line L7 (45.35, 21) -> (45.35, 4)
  line L8 (22.15, 21) -> (4.65, 21)
  line L9 (4.65, 21) -> (4.65, 4)
  line L10 (4.65, 4) -> (22.15, 4)
  line L11 (22.15, 4) -> (22.15, 21)
  constraint horizontal L0
  constraint vertical L1
  constraint horizontal L2
  constraint vertical L3
  constraint horizontal L4
  constraint vertical L5
  constraint horizontal L6
  constraint vertical L7
  constraint horizontal L8
  constraint vertical L9
  constraint horizontal L10
  constraint vertical L11
extrude "Extrude5'" add sketch "Sketch5 (2)" along normal blind 6 from surface at 16.5 separate body makes body 24 in component "Switch_holder"
extrude "Extrude6'" add sketch "Sketch1 (2)" along normal blind 18.5 separate body contours L5 L6 L7 L8 | L12 L13 L14 L15 makes body 25 at (-10.4833, -21, 12.3333) makes body 26 at (-39.5167, -21, 12.3333) in component "Switch_holder"
extrude "Extrude7'" add 2 faces at (-33.6833, -9.6667, 18.5) (-10.4833, -15.3333, 18.5) along direction (0, 0, 1) blind 20 separate body on bodies 25 26 makes body 27 at (-39.5167, -21, 31.8333) makes body 28 at (-10.4833, -21, 31.8333) in component "Switch_holder"
move_face "OffsetFaces1'" offset -0.2 8 faces at (-39.5167, -21, 31.8333) (-45.35, -9.6667, 25.1667) (-33.6833, -4, 25.1667) (-27.85, -15.3333, 25.1667) (-22.15, -15.3333, 25.1667) (-10.4833, -21, 31.8333) (-4.65, -9.6667, 25.1667) (-16.3167, -4, 25.1667) on bodies 27 28 in component "Switch_holder"
move_body "Move1''" bodies 24 to x (1, 0, 0) y (0, 1, 0) z (0, 0, 1) at (0, 0, 4) in component "Switch_holder"
move_face "MoveFace1" by (0, 0, -2) 2 faces at (-53.3333, -16.6667, 23) (3.3333, -16.6667, 23) on bodies 23 in component "Switch_holder"
move_body "Move2'" bodies 24 to x (1, 0, 0) y (0, 1, 0) z (0, 0, 1) at (0, 0, -2) in component "Switch_holder"
sketch "Sketch19" plane through (0, 0, 124) normal (0, 0, 1) x (-1, 0, 0)
  line L0 (10, -5) -> (10, -20)
  line L1 (10, -20) -> (25, -20)
  line L2 (25, -20) -> (25, -100)
  line L3 (25, -100) -> (10, -100)
  line L4 (10, -100) -> (10, -115)
  line L5 (10, -115) -> (25, -115)
  line L6 (25, -115) -> (25, -195)
  line L7 (25, -195) -> (10, -195)
  line L8 (10, -195) -> (10, -210)
  line L9 (10, -210) -> (-49.5, -210)
  line L10 (-49.5, -210) -> (-49.5, -195)
  line L11 (-49.5, -195) -> (-64.5, -195)
  line L12 (-64.5, -195) -> (-64.5, -210)
  line L13 (-64.5, -210) -> (-124, -210)
  line L14 (-124, -210) -> (-124, -195)
  line L15 (-124, -195) -> (-139, -195)
  line L16 (-139, -195) -> (-139, -115)
  line L17 (-139, -115) -> (-124, -115)
  line L18 (-124, -115) -> (-124, -100)
  line L19 (-124, -100) -> (-139, -100)
  line L20 (-139, -100) -> (-139, -20)
  line L21 (-139, -20) -> (-124, -20)
  line L22 (-124, -20) -> (-124, -5)
  line L23 (-124, -5) -> (-64, -5)
  line L24 (-64, -5) -> (-64, -20)
  line L25 (-64, -20) -> (-49, -20)
  line L26 (-49, -20) -> (-49, -5)
  line L27 (-49, -5) -> (10, -5)
  line L28 (30, 0) -> (-138, 0)
  line L29 (-138, 0) -> (-144, 0)
  line L30 (-144, 0) -> (-144, -215)
  line L31 (-144, -215) -> (30, -215)
  line L32 (30, -215) -> (30, 0)
  line L33 (20, 5) -> (35, 5)
  line L34 (35, 5) -> (35, 0)
  line L35 (35, 0) -> (20, 0)
  line L36 (20, 0) -> (20, 5)
  line L37 (35, -10) -> (30, -10)
  line L38 (30, -10) -> (30, 0)
  line L39 (30, 0) -> (35, 0)
  line L40 (35, 0) -> (35, -10)
  constraint horizontal L33
  constraint vertical L34
  constraint horizontal L35
  constraint vertical L36
  constraint horizontal L37
  constraint vertical L38
  constraint horizontal L39
  constraint vertical L40
  constraint coincident L28.start L32.end
extrude "Extrude23" add sketch "Sketch19" against normal blind 60 separate body contours L32 L35 L37 L38 L39 L40 | L28 L33 L34 L35 L36 L39 makes body 29
move_body "Move2''" bodies 29 to x (1, 0, 0) y (0, 1, 0) z (0, 0, 1) at (0, 0, -15)
sketch "Sketch20" plane through (0, 0, 49) normal (0, 0, -1) x (1, 0, 0)
  line L0 (-35, 5) -> (-35, -10)
  line L1 (-35, -10) -> (-30, -10)
  line L2 (-30, -10) -> (-30, 0)
  line L3 (-30, 0) -> (-20, 0)
  line L4 (-20, 0) -> (-20, 5)
  line L5 (-20, 5) -> (-35, 5)
  line L6 (-35, 5) -> (-20, 5)
  line L7 (-20, 5) -> (-20, -10)
  line L8 (-20, -10) -> (-35, -10)
  line L9 (-35, -10) -> (-35, 5)
  constraint horizontal L6
  constraint vertical L7
  constraint horizontal L8
  constraint vertical L9
  constraint coincident L0.start L5.end
extrude "Extrude24" add sketch "Sketch20" along normal blind 5 bodies 29
extrude "Extrude25" add 1 faces at (-33.3333, 1.6667, 109) along direction (0, 0, 1) blind 5 on bodies 29 bodies 29
move_body "Move3'" bodies 22 21 to x (1, 0, 0) y (0, 1, 0) z (0, 0, 1) at (0, 0, -5)
move_body "Move3''" bodies 24 28 23 27 to x (1, 0, 0) y (0, 1, 0) z (0, 0, 1) at (0, 0, -5) in component "Switch_holder"
move_body "Move4'" bodies 21 to x (1, 0, 0) y (0, 1, 0) z (0, 0, 1) at (80, 5, 0)
move_face "OffsetFaces3" offset -15 1 faces at (54, 20, 120) on bodies 20
copy_body "CopyPasteBodies2'" bodies 29 makes body 30
move_body "Move5'" bodies 30 to x (0, -1, 0) y (1, 0, 0) z (0, 0, 1) at (-30, 185, 0)
copy_body "CopyPasteBodies3" bodies 30 makes body 31
move_body "Move6'" bodies 31 to x (0, -1, 0) y (1, 0, 0) z (0, 0, 1) at (-71, 185, 0)
copy_body "CopyPasteBodies4" bodies 31 makes body 32
move_body "Move7'" bodies 32 to x (0, -1, 0) y (1, 0, 0) z (0, 0, 1) at (-71, 144, 0)
sketch "Sketch21" plane through (0, 0, 0) normal (0, 0, -1) x (1, 0, 0)
  line L0 (0, 0) -> (0, -215)
  line L1 (0, -215) -> (114, -215)
  line L2 (114, -215) -> (114, 0)
  line L3 (114, 0) -> (0, 0)
  line L4 (119, -210) -> (109, -210)
  line L5 (109, -210) -> (109, -220)
  line L6 (109, -220) -> (119, -220)
  line L7 (119, -220) -> (119, -210)
  line L8 (119, -210) -> (109, -220) construction
  line L9 (109, -210) -> (119, -220) construction
  line L10 (119, -210) -> (114, -210)
  line L11 (114, -210) -> (114, -205)
  line L12 (114, -205) -> (119, -205)
  line L13 (119, -205) -> (119, -210)
  line L14 (109, -220) -> (104, -220)
  line L15 (104, -220) -> (104, -215)
  line L16 (104, -215) -> (109, -215)
  line L17 (109, -215) -> (109, -220)
  line L18 (119, -220) -> (104, -220)
  line L19 (104, -220) -> (104, -205)
  line L20 (104, -205) -> (119, -205)
  line L21 (119, -205) -> (119, -220)
  point P0 (114, -215)
  dimension "d158" = 10
  dimension "d159" = 10
  constraint horizontal L4
  constraint perpendicular L4 L5
  constraint parallel L4 L6
  constraint parallel L5 L7
  constraint coincident L8 P0
  constraint coincident L9 P0
  constraint coincident P0 L1.end
  constraint horizontal L10
  constraint vertical L11
  constraint horizontal L12
  constraint vertical L13
  constraint coincident L2 L11.end
  constraint horizontal L14
  constraint vertical L15
  constraint horizontal L16
  constraint vertical L17
  constraint coincident L1 L15.end
  constraint horizontal L18
  constraint vertical L19
  constraint horizontal L20
  constraint vertical L21
  measures "d158" distance of L5.end L6.end
  measures "d159" distance of L4.end L5.end
extrude "Extrude26" add sketch "Sketch21" along normal blind 8 separate body contours L1 L2 L4 L5 L11 L16 L19 L20 | L1 L5 L14 L15 L16 L17 L18 L19 | L2 L4 L10 L11 L12 L13 L20 L21 | L1 L2 L4 L5 | L1 L2 L4 L5 L6 L7 L10 L17 L18 L21 makes body 33
extrude "Extrude27" add sketch "Sketch21" against normal blind 20 contours L1 L5 L14 L15 L16 L17 L18 L19 | L2 L4 L10 L11 L12 L13 L20 L21 | L1 L2 L4 L5 L6 L7 L10 L17 L18 L21 bodies 33
copy_body "CopyPasteBodies5" bodies 33 makes body 34
move_body "Move8" bodies 34 to x (0, 1, 0) y (-1, 0, 0) z (0, 0, 1) at (215, 101, 0)
copy_body "CopyPasteBodies6" bodies 34 makes body 35
move_body "Move9" bodies 35 to x (0, 1, 0) y (-1, 0, 0) z (0, 0, 1) at (215, 0, 0)
copy_body "CopyPasteBodies7" bodies 35 makes body 36
move_body "Move10" bodies 36 to x (0, 1, 0) y (-1, 0, 0) z (0, 0, 1) at (114, 0, 0)
component "Alimentatore" placed x (1, 0, 0) y (0, 1, 0) z (0, 0, 1) at (0, 0, 0)
component "Relays" placed x (1, 0, 0) y (0, 1, 0) z (0, 0, 1) at (-20, 10, 55)
component "Buck_conv" placed x (0, 1, 0) y (-1, 0, 0) z (0, 0, 1) at (138, 177, 55)
component "Breadbord" placed x (0, -1, 0) y (1, 0, 0) z (0, 0, 1) at (84, 173, 55)
component "Arduino" placed x (1, 0, 0) y (0, 1, 0) z (0, 0, 1) at (80, 0, 70)
component "Mosfet" placed x (-1, 0, 0) y (0, -1, 0) z (0, 0, 1) at (58, 180, 55)